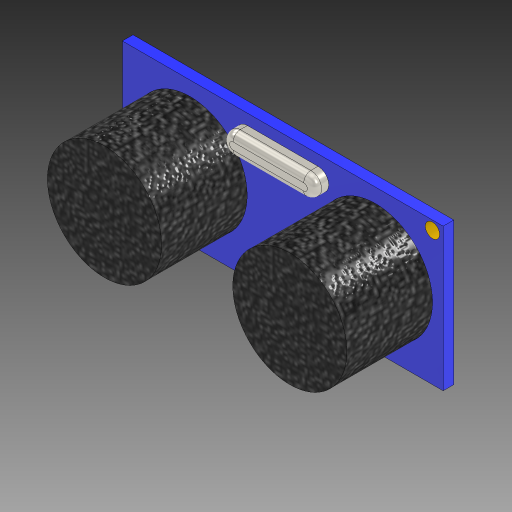
# Autodesk Inventor part: UltraZvuk
Saved by Autodesk Inventor 2023 (Build 270158000, 158)
## iProperties
Created: 2024-02-02
Part Number: UltraZvuk
Material: Všeobecné
Document SubType Name: Modeling
Designer: matej
Mass: 6.38965 g
Surface Area: 35.1113 cm^2
Volume: 6.38965 cm^3
Density: 1 g/cm^3
Appearance: Modrá – nástěnná malba – lesklá
Author: matej
Autodesk Inventor part; units mm, degrees
ref_plane "YZ Plane" through (0, 0, 0) normal (1, 0, 0) x (0, 1, 0)
ref_plane "XZ Plane" through (0, 0, 0) normal (0, 1, 0) x (-1, 0, 0)
ref_plane "XY Plane" through (0, 0, 0) normal (0, 0, 1) x (1, 0, 0)
sketch "Náčrt1" plane through (0, 0, 0) normal (0, 0, 1) x (1, 0, 0)
  line L0 (-22.5, -10) -> (22.5, -10)
  line L1 (22.5, -10) -> (22.5, 10)
  line L2 (22.5, 10) -> (-22.5, 10)
  line L3 (-22.5, 10) -> (-22.5, -10)
  line L4 (-22.5, -10) -> (22.5, 10) construction
  line L5 (22.5, -10) -> (-22.5, 10) construction
  point P0 (0, 0)
  dimension "d0" = 45
  dimension "d1" = 20
  constraints: 12 end point, 2 midpoint, 2 parallel, 1 horizontal, 1 perpendicular
  measures "d0" distance of L2.end L1.end
  measures "d1" distance of L1.end L0.end
extrude "Vysunutí1" add sketch "Náčrt1" along normal blind 1.5
sketch "Náčrt2" plane through (0, 0, 1.5) normal (0, 0, 1) x (1, 0, 0)
  circle A0 centre (13, 0) radius 8
  circle A1 centre (-13, 0) radius 8
  point P0 (0, 0)
  dimension "d4" = 16
  dimension "d5" = 16
  dimension "d6" = 26
  dimension "d7" = 13
  constraints: 2 centre point
  measures "d4" diameter of A0
  measures "d5" diameter of A1
  measures "d6" distance of A0.centre A1.centre
  measures "d7" distance of point (0, 0) A0.centre
extrude "Vysunutí2" add sketch "Náčrt2" along normal blind 12
sketch "Náčrt3" plane through (0, 0, 1.5) normal (0, 0, 1) x (1, 0, 0)
  line L0 (-4.9518, 7) -> (4.9518, 7) construction
  line L1 (-4.9518, 5.5) -> (4.9518, 5.5)
  line L2 (4.9518, 8.5) -> (-4.9518, 8.5)
  arc A0 (-4.9518, 8.5) -> (-4.9518, 5.5) centre (-4.9518, 7) ccw
  arc A1 (4.9518, 5.5) -> (4.9518, 8.5) centre (4.9518, 7) ccw
  point P0 (0, 0)
  point P1 (0, 7)
  dimension "d10" = 3
  dimension "d11" = 7
  constraints: 8 end point, 4 point on circle, 4 tangent, 2 centre point, 1 horizontal, 1 midpoint, 1 parallel
  measures "d10" diameter of A1
  measures "d11" distance of point (0, 0) point (0, 7)
extrude "Vysunutí3" add sketch "Náčrt3" along normal blind 2
fillet "Zaoblení1" radius 1 4 edges at (0, 8.5, 3.5) (-6.4518, 7, 3.5) (0, 5.5, 3.5) (6.4518, 7, 3.5)
sketch "Náčrt4" plane through (0, 0, 1.5) normal (0, 0, 1) x (1, 0, 0)
  circle A0 centre (21, 8.75) radius 1
  circle A1 centre (-21, -8.75) radius 1
  point P0 (0, 0)
  dimension "d15" = 2
  dimension "d16" = 2
  dimension "d17" = 17.5
  dimension "d18" = 42
  dimension "d19" = 8.75
  dimension "d20" = 21
  constraints: 2 centre point
  measures "d15" diameter of A0
  measures "d16" diameter of A1
  measures "d17" vertical distance of A0.centre A1.centre
  measures "d18" horizontal distance of A0.centre A1.centre
  measures "d19" vertical distance of point (0, 0) A1.centre
  measures "d20" horizontal distance of point (0, 0) A0.centre
extrude "Vysunutí4" cut sketch "Náčrt4" against normal through all
sketch "Náčrt6" plane through (0, 0, 0) normal (1, 0, 0) x (0, 1, 0)
  line L0 (-10, 0) -> (10, 0) projected
  line L1 (-10, 0) -> (-8, 0)
  line L2 (-8, 0) -> (-8, -2)
  line L3 (-8, -2) -> (-10, -2)
  line L4 (-10, -2) -> (-10, 0)
  line L5 (-8, -2) -> (-16, -2)
  line L6 (-16, -2) -> (-16, -3)
  line L7 (-16, -3) -> (-8, -3)
  line L8 (-8, -3) -> (-8, -2)
  point P0 (0, 0)
  dimension "d23" = 2
  dimension "d24" = 2
  dimension "d25" = 8
  dimension "d26" = 1
  constraints: 16 end point, 4 parallel, 2 horizontal, 2 perpendicular
  measures "d23" distance of L2.end L3.end
  measures "d24" distance of L1.end L2.end
  measures "d25" distance of L7.end L6.end
  measures "d26" distance of L6.end L5.end
extrude "Vysunutí5" add sketch "Náčrt6" along normal mid plane 13
